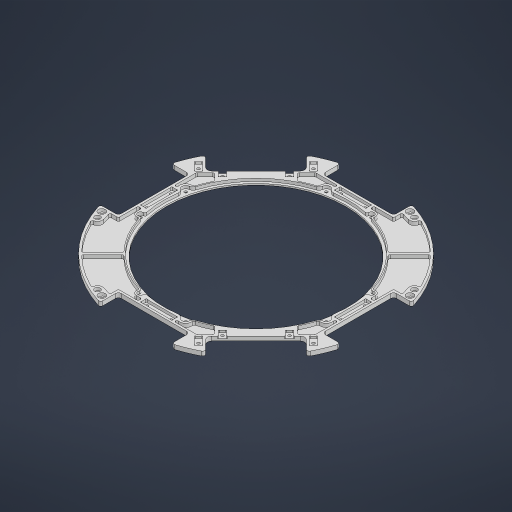
# Autodesk Inventor part: BasePlate
Saved by Autodesk Inventor 2024.2 (Build 282272000, 272)
## iProperties
Created: 2023-12-21
Part Number: BasePlate
Material: 一般
Document SubType Name: Modeling
Designer: Hanaoka
Density: 1 g/cm^3
Appearance: 既定
Author: Hanaoka
Autodesk Inventor part; units mm, degrees
ref_plane "YZ Plane" through (0, 0, 0) normal (1, 0, 0) x (0, 1, 0)
ref_plane "XZ Plane" through (0, 0, 0) normal (0, 1, 0) x (-1, 0, 0)
ref_plane "XY Plane" through (0, 0, 0) normal (0, 0, 1) x (1, 0, 0)
derived "MotorMount_main.ipt"
sketch "スケッチ4" plane through (-11, -15, 0) normal (0, -1, 0) x (1, 0, 0)
  circle A0 centre (19.5, 2) radius 0.8 projected
  circle A1 centre (2.5, 2) radius 0.8 projected
  line L0 (22, 0) -> (0, 0) projected
  line L1 (0, 0) -> (0, 4) projected
  line L2 (22, 4) -> (0, 4) projected
  line L3 (22, 0) -> (22, 4) projected
  circle A2 centre (11, -66) radius 90 construction
  line L4 (2.5, 2) -> (19.5, 2) construction
  line L5 (11, 2) -> (11, -66) construction
  circle A3 centre (11, -66) radius 88
  line L6 (-14, 18.3742) -> (-14, 7.5)
  line L7 (-12, 5.5) -> (34, 5.5)
  line L8 (36, 7.5) -> (36, 18.3742)
  arc A4 (-14, 7.5) -> (-12, 5.5) centre (-12, 7.5) ccw
  arc A5 (34, 5.5) -> (36, 7.5) centre (34, 7.5) ccw
  line L9 (0, 0) -> (22, 0)
  line L10 (22, 0) -> (22, 4)
  line L11 (22, 4) -> (0, 4)
  line L12 (0, 4) -> (0, 0)
  circle A6 centre (19.5, 2) radius 1
  circle A7 centre (2.5, 2) radius 1
  circle A8 centre (-57, -74.5) radius 1
  line L13 (-59, -77) -> (-55, -77)
  line L14 (-57, -74.5) -> (-57, -57.5) construction
  line L15 (-59, -55) -> (-59, -77)
  line L16 (-55, -55) -> (-59, -55)
  line L17 (-55, -77) -> (-55, -55)
  line L18 (-60.5, -89) -> (-60.5, -43)
  circle A9 centre (-57, -57.5) radius 1
  arc A10 (-62.5, -91) -> (-60.5, -89) centre (-62.5, -89) ccw
  line L19 (-62.5, -41) -> (-73.3742, -41)
  arc A11 (-60.5, -43) -> (-62.5, -41) centre (-62.5, -43) ccw
  line L20 (-73.3742, -91) -> (-62.5, -91)
  circle A12 centre (19.5, -134) radius 1
  line L21 (22, -136) -> (22, -132)
  line L22 (19.5, -134) -> (2.5, -134) construction
  line L23 (0, -136) -> (22, -136)
  line L24 (0, -132) -> (0, -136)
  line L25 (22, -132) -> (0, -132)
  line L26 (34, -137.5) -> (-12, -137.5)
  circle A13 centre (2.5, -134) radius 1
  arc A14 (36, -139.5) -> (34, -137.5) centre (34, -139.5) ccw
  line L27 (-14, -139.5) -> (-14, -150.3742)
  arc A15 (-12, -137.5) -> (-14, -139.5) centre (-12, -139.5) ccw
  line L28 (36, -150.3742) -> (36, -139.5)
  circle A16 centre (79, -57.5) radius 1
  line L29 (81, -55) -> (77, -55)
  line L30 (79, -57.5) -> (79, -74.5) construction
  line L31 (81, -77) -> (81, -55)
  line L32 (77, -77) -> (81, -77)
  line L33 (77, -55) -> (77, -77)
  line L34 (82.5, -43) -> (82.5, -89)
  circle A17 centre (79, -74.5) radius 1
  arc A18 (84.5, -41) -> (82.5, -43) centre (84.5, -43) ccw
  line L35 (84.5, -91) -> (95.3742, -91)
  arc A19 (82.5, -89) -> (84.5, -91) centre (84.5, -89) ccw
  line L36 (95.3742, -41) -> (84.5, -41)
  arc A20 (77.7071, -55) -> (77, -55.7071) centre (77.3536, -55.3536) ccw
  line L37 (77.3536, -55.3536) -> (77.3536, -55) construction
  line L38 (77.3536, -55.3536) -> (77, -55.3536) construction
  line L39 (77.3536, -55.3536) -> (77, -55) construction
  line L40 (80.6464, -55) -> (80.6464, -55.3536) construction
  line L41 (80.6464, -55.3536) -> (81, -55.3536) construction
  line L42 (77.3536, -77) -> (77.3536, -76.6464) construction
  line L43 (77.3536, -76.6464) -> (77, -76.6464) construction
  line L44 (81, -76.6464) -> (80.6464, -76.6464) construction
  line L45 (80.6464, -76.6464) -> (80.6464, -77) construction
  line L46 (81, -77) -> (80.6464, -76.6464) construction
  line L47 (77.3536, -76.6464) -> (77, -77) construction
  line L48 (81, -55) -> (80.6464, -55.3536) construction
  arc A21 (81, -55.7071) -> (80.2929, -55) centre (80.6464, -55.3536) ccw
  arc A22 (80.2929, -77) -> (81, -76.2929) centre (80.6464, -76.6464) ccw
  arc A23 (77, -76.2929) -> (77.7071, -77) centre (77.3536, -76.6464) ccw
  arc A24 (21.2929, 0) -> (22, 0.7071) centre (21.6464, 0.3536) ccw
  arc A25 (22, 3.2929) -> (21.2929, 4) centre (21.6464, 3.6464) ccw
  arc A26 (0, 0.7071) -> (0.7071, 0) centre (0.3536, 0.3536) ccw
  arc A27 (0.7071, 4) -> (0, 3.2929) centre (0.3536, 3.6464) ccw
  arc A28 (-55, -55.7071) -> (-55.7071, -55) centre (-55.3536, -55.3536) ccw
  arc A29 (-58.2929, -55) -> (-59, -55.7071) centre (-58.6464, -55.3536) ccw
  arc A30 (-55.7071, -77) -> (-55, -76.2929) centre (-55.3536, -76.6464) ccw
  arc A31 (-59, -76.2929) -> (-58.2929, -77) centre (-58.6464, -76.6464) ccw
  arc A32 (0.7071, -132) -> (0, -132.7071) centre (0.3536, -132.3536) ccw
  arc A33 (0, -135.2929) -> (0.7071, -136) centre (0.3536, -135.6464) ccw
  arc A34 (22, -132.7071) -> (21.2929, -132) centre (21.6464, -132.3536) ccw
  arc A35 (21.2929, -136) -> (22, -135.2929) centre (21.6464, -135.6464) ccw
  point P0 (11, 0)
  point P1 (-14, 5.5)
  point P2 (36, 5.5)
  point P3 (-57, -66)
  point P4 (-60.5, -91)
  point P5 (-60.5, -41)
  point P6 (11, -134)
  point P7 (36, -137.5)
  point P8 (-14, -137.5)
  point P9 (79, -66)
  point P10 (82.5, -41)
  point P11 (82.5, -91)
  point P12 (22, -135.2929)
  point P13 (21.2929, -136)
  point P14 (0.7071, -136)
  point P15 (0, -135.2929)
  point P16 (0, -132.7071)
  point P17 (0.7071, -132)
  point P18 (21.2929, -132)
  point P19 (22, -132.7071)
  point P20 (-58.2929, -77)
  point P21 (-59, -76.2929)
  point P22 (-59, -55.7071)
  point P23 (-58.2929, -55)
  point P24 (-55.7071, -55)
  point P25 (-55, -55.7071)
  point P26 (-55, -76.2929)
  point P27 (-55.7071, -77)
  point P28 (0, 3.2929)
  point P29 (0.7071, 4)
  point P30 (21.2929, 4)
  point P31 (22, 3.2929)
  point P32 (22, 0.7071)
  point P33 (21.2929, 0)
  point P34 (0.7071, 0)
  point P35 (0, 0.7071)
  dimension "d4" = 180
  dimension "d5" = 68
  dimension "d6" = 176
  dimension "d11" = 1.5
  dimension "d12" = 50
  dimension "d13" = 2
  dimension "d14" = 2
  dimension "d17" = 360
  dimension "d31" = 0.5
  dimension "d32" = 0.5
  dimension "d35" = 360
  constraints: 90 end point, 50 point on circle, 34 centre point, 32 point on line, 13 coincident, 8 equal length, 6 perpendicular, 5 equal radius, 4 horizontal, 4 tangent, 4 vertical, 3 parallel, 1 midpoint, 190 other
  measures "d4" diameter of A2
  measures "d5" distance of L5.start L5.end
  measures "d6" diameter of A3
  measures "d11" distance between parallel lines of L7 L2
  measures "d12" distance of point (-14, 5.5) point (36, 5.5)
  measures "d13" radius of A4
  measures "d14" diameter of A7
  measures "d31" radius of A20
  measures "d32" distance of L37.start L29.end
extrude "押し出し2" add sketch "スケッチ4" along normal blind 1 contours A24 L0 | L0 L1 L2 L3 | L3 A24 | A26 L0 | L3 A25 | A26 L1 | L2 A25 | A27 L1 | L2 A27 | L36 A18 L34 A19 L35 A3 L28 A14 L26 A15 L27 L20 A10 L18 A11 L19 L6 A4 L7 A5 L8 | L15 L16 L17 L13 | A31 L15 | L13 A31 | L13 A30 | A29 L15 | L17 A30 | A29 L16 | L17 A28 | A28 L16 | L23 L24 L25 L21 | A35 L23 | L21 A35 | L21 A34 | A33 L23 | L25 A34 | A33 L24 | L25 A32 | A32 L24 | L31 L32 L33 L29 | A21 L31 | L29 A21 | L29 A20 | A22 L31 | L33 A20 | A22 L32 | L33 A23 | A23 L32
extrude "押し出し3" add sketch "スケッチ4" against normal blind 2 contours L36 A18 L34 A19 L35 A3 L28 A14 L26 A15 L27 L20 A10 L18 A11 L19 L6 A4 L7 A5 L8
fillet "フィレット1" radius 1.5 8 edges at (-84.3742, -14.5, -41) (-25, -14.5, 18.3742) (25, -14.5, 18.3742) (84.3742, -14.5, -41) (84.3742, -14.5, -91) (25, -14.5, -150.3742) (-25, -14.5, -150.3742) (-84.3742, -14.5, -91)
sketch "溝切り" plane through (-23, -13, 5.5) normal (0, 1, 0) x (1, 0, 0)
  circle A0 centre (102.5487, 100) radius 2.5
  line L0 (96.5, 96.5) -> (105.3408, 96.5) projected
  arc A1 (106.7686, 98.4595) -> (49.9595, 155.2686) centre (23, 71.5) ccw projected
  circle A2 centre (102.5487, 100) radius 3.5 construction
  line L1 (85.2254, 133.7254) -> (-39.2254, 9.2746) construction
  arc A3 (-60.7686, 44.5405) -> (-3.9595, -12.2686) centre (23, 71.5) ccw projected
  circle A4 centre (51.5, 151.0487) radius 2.5
  circle A5 centre (51.5, 151.0487) radius 3.5 construction
  line L2 (-39.2254, 133.7254) -> (85.2254, 9.2746) construction
  arc A6 (49.9595, -12.2686) -> (106.7686, 44.5405) centre (23, 71.5) ccw projected
  arc A7 (-3.9595, 155.2686) -> (-60.7686, 98.4595) centre (23, 71.5) ccw projected
  circle A8 centre (-5.5, -8.0487) radius 2.5
  circle A9 centre (-5.5, -8.0487) radius 3.5 construction
  circle A10 centre (-56.5487, 43) radius 3.5 construction
  circle A11 centre (-56.5487, 43) radius 2.5
  circle A12 centre (102.5487, 100) radius 1.3
  circle A13 centre (51.5, 151.0487) radius 1.3
  circle A14 centre (-56.5487, 43) radius 1.3
  circle A15 centre (-5.5, -8.0487) radius 1.3
  circle A16 centre (23, 71.5) radius 63
  line L3 (-54.3392, 113.4839) -> (-46.9146, 106.0593)
  line L4 (-42.672, 106.0593) -> (-11.5593, 137.172)
  line L5 (-11.5593, 141.4146) -> (-18.9839, 148.8392)
  arc A17 (-46.9146, 106.0593) -> (-42.672, 106.0593) centre (-44.7933, 108.1806) ccw
  arc A18 (-11.5593, 137.172) -> (-11.5593, 141.4146) centre (-13.6806, 139.2933) ccw
  circle A19 centre (-41.9648, 136.4648) radius 21 construction
  line L6 (64.9839, -5.8392) -> (57.5593, 1.5854)
  line L7 (57.5593, 5.828) -> (88.672, 36.9407)
  line L8 (92.9146, 36.9407) -> (100.3392, 29.5161)
  arc A20 (57.5593, 5.828) -> (57.5593, 1.5854) centre (59.6806, 3.7067) ccw
  arc A21 (92.9146, 36.9407) -> (88.672, 36.9407) centre (90.7933, 34.8194) ccw
  circle A22 centre (8.2095, 135.5648) radius 2.75 construction
  circle A23 centre (8.2095, 135.5648) radius 1
  line L9 (8.2095, 135.5648) -> (23, 71.5) construction
  arc A24 (10.889, 136.1834) -> (5.53, 134.9462) centre (8.2095, 135.5648) ccw
  line L10 (5.53, 134.9462) -> (6.1621, 132.2082)
  line L11 (10.889, 136.1834) -> (11.5211, 133.4454)
  circle A25 centre (-41.0648, 86.2905) radius 2.75 construction
  circle A26 centre (-41.0648, 86.2905) radius 1
  arc A27 (-40.4462, 88.97) -> (-41.6834, 83.611) centre (-41.0648, 86.2905) ccw
  line L12 (-40.4462, 88.97) -> (-37.7082, 88.3379)
  line L13 (-41.6834, 83.611) -> (-38.9454, 82.9789)
  circle A28 centre (87.0648, 56.7095) radius 2.75 construction
  circle A29 centre (87.0648, 56.7095) radius 1
  arc A30 (86.4462, 54.03) -> (87.6834, 59.389) centre (87.0648, 56.7095) ccw
  line L14 (86.4462, 54.03) -> (83.7082, 54.6621)
  line L15 (87.6834, 59.389) -> (84.9454, 60.0211)
  line L16 (35.111, 6.8166) -> (34.4789, 9.5546)
  line L17 (40.47, 8.0538) -> (39.8379, 10.7918)
  circle A31 centre (37.7905, 7.4352) radius 2.75 construction
  circle A32 centre (37.7905, 7.4352) radius 1
  arc A33 (35.111, 6.8166) -> (40.47, 8.0538) centre (37.7905, 7.4352) ccw
  circle A34 centre (23, 71.5) radius 64
  line L18 (-48.5, 94.5) -> (-48.5, 96.331) construction
  line L19 (-48.5, 96.331) -> (-58.019, 105.85) construction
  line L20 (-48.5, 94.5) -> (-48.5, 48.5) projected
  line L21 (0, 143) -> (-1.831, 143) construction
  line L22 (-1.831, 143) -> (-11.35, 152.519) construction
  arc A35 (-60.7686, 98.4595) -> (-59.3408, 96.5) centre (-59.3408, 98) ccw projected
  line L23 (-59.3408, 96.5) -> (-50.5, 96.5) projected
  arc A36 (-48.5, 94.5) -> (-50.5, 96.5) centre (-50.5, 94.5) ccw projected
  arc A37 (-2, 153.8408) -> (-3.9595, 155.2686) centre (-3.5, 153.8408) ccw projected
  line L24 (-2, 145) -> (-2, 153.8408) projected
  arc A38 (-2, 145) -> (0, 143) centre (0, 145) ccw projected
  line L25 (46, 143) -> (0, 143) projected
  point P0 (23, 5.5)
  point P1 (-44.7933, 103.9379)
  point P2 (-9.4379, 139.2933)
  point P3 (100.3392, 29.5161)
  point P4 (39.8379, 10.7918)
  point P5 (34.4789, 9.5546)
  point P6 (84.9454, 60.0211)
  point P7 (83.7082, 54.6621)
  point P8 (-38.9454, 82.9789)
  point P9 (-37.7082, 88.3379)
  point P10 (-39.9207, 83.2041)
  point P11 (34.7041, 8.5793)
  point P12 (40.0631, 9.8165)
  point P13 (84.6835, 54.4369)
  point P14 (85.9207, 59.7959)
  point P15 (11.2959, 134.4207)
  point P16 (5.9369, 133.1835)
  point P17 (-38.6835, 88.5631)
  point P18 (-50.6269, 109.7716)
  point P19 (-11.35, 152.519)
  dimension "d20" = 5
  dimension "d22" = 7
  dimension "d23" = 2.6
  dimension "d37" = 50
  dimension "d38" = 3
  dimension "d39" = 42
  dimension "d40" = 13.5
  dimension "d45" = 2
  dimension "d46" = 5.5
  dimension "d47" = 32
  dimension "d102" = 8
  dimension "d106" = 126
  dimension "d107" = 1
  constraints: 42 end point, 38 symmetric about line, 31 centre point, 25 point on circle, 18 coincident, 11 tangent, 7 parallel, 5 equal radius, 5 point on line, 2 midpoint, 1 collinear, 1 vertical, 17 other
  measures "d20" diameter of A0
  measures "d22" diameter of A2
  measures "d23" diameter of A12
  measures "d37" distance of point (-44.793, 103.938) point (-9.438, 139.293)
  measures "d38" radius of A17
  measures "d39" diameter of A19
  measures "d40" distance from line of L5.end L4
  measures "d45" diameter of A23
  measures "d46" diameter of A22
  measures "d47" angle of L2 L9
  measures "d102" distance from line of point (-50.627, 109.772) L19
  measures "d106" diameter of A16
  measures "d107" radial gap between concentric circles of A16 A34
extrude "押し出し4" cut sketch "溝切り" against normal up to surface (3 mm away) contours A12 | A13 | A14 | A15
extrude "押し出し5" cut sketch "溝切り" against normal blind 2 contours A0 | A4 | A8 | A11 | A15 | A16 | A16 L11 A34 L15 | A16 L10 A34 L11 | L15 A34 L14 A16 | A16 L12 A34 L10 | A34 L10 A24 L11 | L14 A34 L17 A16 | L15 A30 L14 A34 | A16 L13 A34 L12 | L17 A34 L16 A16 | A16 L16 A34 L13 | A34 L13 A27 L12 | L17 A33 L16 A34
extrude "押し出し6" cut sketch "溝切り" against normal up to surface (3 mm away) contours L6 A20 L7 A21 L8 A6 | L5 A18 L4 A17 L3 A7 | A16 | A23 | A26 | A29 | A32
fillet "フィレット2" radius 1.5 12 edges at (-77.3392, -14.5, -107.9839) (-41.9839, -14.5, -143.3392) (41.9839, -14.5, 11.3392) (77.3392, -14.5, -24.0161) (-62.9207, -14, -77.7041) (-61.6835, -14, -83.0631) (11.7041, -14, -3.0793) (17.0631, -14, -4.3165) (61.6835, -14, -48.9369) (62.9207, -14, -54.2959) (-17.0631, -14, -127.6835) (-11.7041, -14, -128.9207)
sketch "シャフト用はめ穴" plane through (-23, -13, -137.5) normal (0, 1, 0) x (1, 0, 0)
  circle A0 centre (-54.5262, -105.1146) radius 1
  circle A1 centre (-54.5262, -105.1146) radius 2
  circle A2 centre (-41.4205, -88) radius 2
  circle A3 centre (-41.4205, -88) radius 1
  circle A4 centre (-56.5487, -100) radius 2.5 projected
  circle A5 centre (23, -71.5) radius 63 projected
  arc A6 (-56.5487, -100) -> (-54.5262, -105.1146) centre (23, -71.5) ccw construction
  line L0 (85.2254, -9.2746) -> (-39.2254, -133.7254) construction
  line L1 (-39.2254, -9.2746) -> (85.2254, -133.7254) construction
  circle A7 centre (-10.6146, -149.0262) radius 1
  circle A8 centre (-10.6146, -149.0262) radius 2
  circle A9 centre (-41.4205, -88) radius 2.5 construction
  arc A10 (5.9369, -9.8165) -> (-38.6835, -54.4369) centre (23, -71.5) ccw projected
  line L2 (-43.7071, -82.5) -> (-46.2929, -82.5) projected
  circle A11 centre (6.5, -135.9205) radius 2
  circle A12 centre (6.5, -135.9205) radius 1
  circle A13 centre (6.5, -135.9205) radius 2.5 construction
  circle A14 centre (56.6146, 6.0262) radius 1
  circle A15 centre (56.6146, 6.0262) radius 2
  circle A16 centre (39.5, -7.0795) radius 2
  circle A17 centre (39.5, -7.0795) radius 1
  circle A18 centre (100.5262, -37.8854) radius 1
  circle A19 centre (100.5262, -37.8854) radius 2
  circle A20 centre (87.4205, -55) radius 2
  circle A21 centre (87.4205, -55) radius 1
  line L3 (23, -71.5) -> (-41.4205, -88) construction
  point P0 (23, -137.5)
  point P1 (33.5618, -134.6225)
  point P2 (-40.1225, -60.9382)
  dimension "d50" = 2
  dimension "d51" = 4
  dimension "d52" = 1
  dimension "d53" = 5
  dimension "d54" = 3
  constraints: 19 centre point, 13 symmetric about line, 12 coincident, 2 end point, 2 equal radius, 2 midpoint, 2 point on circle, 1 tangent, 13 other
  measures "d50" diameter of A0
  measures "d51" diameter of A1
  measures "d53" diameter of A9
  measures "d54" distance edge to line of A9 L2
extrude "押し出し7" cut sketch "シャフト用はめ穴" against normal up to surface (2 mm away) contours A0 | A1 | A2 | A3 | A7 | A8 | A11 | A12 | A14 | A15 | A16 | A17 | A18 | A19 | A20 | A21
extrude "押し出し8" cut sketch "シャフト用はめ穴" against normal up to surface (3 mm away) contours A0 | A3 | A7 | A12 | A14 | A17 | A18 | A21
sketch "キッカー用はめあい" plane through (-23, -13, -137.5) normal (0, 1, 0) x (1, 0, 0)
  circle A0 centre (83.1212, -108.0745) radius 1
  circle A1 centre (59.5745, -131.6212) radius 1
  line L0 (88.672, -106.0593) -> (57.5593, -137.172) projected
  line L1 (73.1156, -121.6156) -> (68.2548, -116.7548) construction
  line L2 (57.5593, -137.172) -> (88.672, -106.0593) projected
  arc A2 (5.9369, -9.8165) -> (-38.6835, -54.4369) centre (23, -71.5) ccw projected
  line L3 (59.5745, -131.6212) -> (83.1212, -108.0745) construction
  line L4 (86.3031, -108.4281) -> (82.7676, -104.8925)
  line L5 (82.7676, -104.8925) -> (79.9392, -107.721)
  line L6 (79.9392, -107.721) -> (83.4747, -111.2565)
  circle A3 centre (83.1212, -108.0745) radius 2 construction
  line L7 (59.9281, -134.8031) -> (56.3925, -131.2676)
  line L8 (56.3925, -131.2676) -> (59.221, -128.4392)
  line L9 (59.221, -128.4392) -> (62.7565, -131.9747)
  line L10 (82.7676, -104.8925) -> (83.1212, -105.2461)
  line L11 (79.9392, -107.721) -> (80.2927, -108.0745)
  line L12 (-21.5477, -116.0477) -> (67.5477, -26.9523) construction
  circle A4 centre (23, -71.5) radius 63 projected
  circle A5 centre (-13.5745, -11.3788) radius 1
  circle A6 centre (-37.1212, -34.9255) radius 1
  line L13 (-27.1156, -21.3844) -> (-22.2548, -26.2452) construction
  line L14 (-37.1212, -34.9255) -> (-13.5745, -11.3788) construction
  line L15 (-13.9281, -8.1969) -> (-10.3925, -11.7324)
  line L16 (-10.3925, -11.7324) -> (-13.221, -14.5608)
  line L17 (-13.221, -14.5608) -> (-16.7565, -11.0253)
  circle A7 centre (-13.5745, -11.3788) radius 2 construction
  line L18 (-40.3031, -34.5719) -> (-36.7676, -38.1075)
  line L19 (-36.7676, -38.1075) -> (-33.9392, -35.279)
  line L20 (-33.9392, -35.279) -> (-37.4747, -31.7435)
  line L21 (-10.3925, -11.7324) -> (-10.7461, -11.3788)
  line L22 (-13.221, -14.5608) -> (-13.5745, -14.2073)
  line L23 (-40.3031, -34.5719) -> (-37.4747, -31.7435)
  line L24 (-42.672, -36.9407) -> (-11.5593, -5.828) projected
  line L25 (-16.7565, -11.0253) -> (-13.9281, -8.1969)
  line L26 (-54.3392, -37.2943) -> (-51.5108, -34.4659)
  line L27 (-51.5108, -34.4659) -> (-45.8539, -40.1227)
  line L28 (-45.8539, -40.1227) -> (-48.6824, -42.9512)
  line L29 (-48.6824, -42.9512) -> (-54.3392, -37.2943)
  line L30 (-46.9146, -36.9407) -> (-52.9014, -30.954) projected
  line L31 (-11.5593, -5.828) -> (-42.672, -36.9407) projected
  circle A8 centre (-50.0966, -38.7085) radius 1
  line L32 (-51.5108, -40.1227) -> (-48.6824, -37.2943) construction
  line L33 (-47.2681, -41.5369) -> (-52.925, -35.8801) construction
  arc A9 (-53.8392, -36.7943) -> (-53.8392, -37.7943) centre (-53.8392, -37.2943) ccw
  line L34 (-54.3392, -37.2943) -> (-53.8392, -37.2943) construction
  line L35 (-53.8392, -37.2943) -> (-54.0892, -37.0443) construction
  line L36 (-53.8392, -37.2943) -> (-54.0892, -37.5443) construction
  arc A10 (-51.0108, -34.9659) -> (-52.0108, -34.9659) centre (-51.5108, -34.9659) ccw
  arc A11 (-49.1824, -42.4512) -> (-48.1824, -42.4512) centre (-48.6824, -42.4512) ccw
  arc A12 (-46.3539, -40.6227) -> (-46.3539, -39.6227) centre (-46.3539, -40.1227) ccw
  line L37 (-11.2057, 5.8392) -> (-14.0341, 3.0108)
  line L38 (-14.0341, 3.0108) -> (-8.3773, -2.6461)
  line L39 (-8.3773, -2.6461) -> (-5.5488, 0.1824)
  line L40 (-5.5488, 0.1824) -> (-11.2057, 5.8392)
  circle A13 centre (-9.7915, 1.5966) radius 1
  arc A14 (-10.7057, 5.3392) -> (-11.7057, 5.3392) centre (-11.2057, 5.3392) ccw
  arc A15 (-13.5341, 3.5108) -> (-13.5341, 2.5108) centre (-13.5341, 3.0108) ccw
  arc A16 (-6.0488, -0.3176) -> (-6.0488, 0.6824) centre (-6.0488, 0.1824) ccw
  arc A17 (-8.8773, -2.1461) -> (-7.8773, -2.1461) centre (-8.3773, -2.1461) ccw
  line L41 (57.2057, -148.8392) -> (60.0341, -146.0108)
  line L42 (60.0341, -146.0108) -> (54.3773, -140.3539)
  line L43 (54.3773, -140.3539) -> (51.5488, -143.1824)
  line L44 (51.5488, -143.1824) -> (57.2057, -148.8392)
  circle A18 centre (55.7915, -144.5966) radius 1
  arc A19 (56.7057, -148.3392) -> (57.7057, -148.3392) centre (57.2057, -148.3392) ccw
  arc A20 (59.5341, -146.5108) -> (59.5341, -145.5108) centre (59.5341, -146.0108) ccw
  arc A21 (52.0488, -142.6824) -> (52.0488, -143.6824) centre (52.0488, -143.1824) ccw
  arc A22 (54.8773, -140.8539) -> (53.8773, -140.8539) centre (54.3773, -140.8539) ccw
  line L45 (94.6824, -100.0488) -> (100.3392, -105.7057)
  arc A23 (99.8392, -106.2057) -> (99.8392, -105.2057) centre (99.8392, -105.7057) ccw
  line L46 (100.3392, -105.7057) -> (97.5108, -108.5341)
  arc A24 (97.0108, -108.0341) -> (98.0108, -108.0341) centre (97.5108, -108.0341) ccw
  line L47 (97.5108, -108.5341) -> (91.8539, -102.8773)
  circle A25 centre (96.0966, -104.2915) radius 1
  line L48 (91.8539, -102.8773) -> (94.6824, -100.0488)
  arc A26 (95.1824, -100.5488) -> (94.1824, -100.5488) centre (94.6824, -100.5488) ccw
  arc A27 (92.3539, -102.3773) -> (92.3539, -103.3773) centre (92.3539, -102.8773) ccw
  arc A28 (83.2676, -105.3925) -> (82.2676, -105.3925) centre (82.7676, -105.3925) ccw
  line L49 (82.5176, -105.1425) -> (82.7676, -105.3925) construction
  line L50 (82.7676, -105.3925) -> (83.0176, -105.1425) construction
  line L51 (82.7676, -105.3925) -> (82.7676, -104.8925) construction
  line L52 (80.1892, -107.971) -> (80.4392, -107.721) construction
  line L53 (80.4392, -107.721) -> (80.1892, -107.471) construction
  line L54 (80.4392, -107.721) -> (79.9392, -107.721) construction
  arc A29 (80.4392, -107.221) -> (80.4392, -108.221) centre (80.4392, -107.721) ccw
  arc A30 (56.8925, -130.7676) -> (56.8925, -131.7676) centre (56.8925, -131.2676) ccw
  arc A31 (59.721, -128.9392) -> (58.721, -128.9392) centre (59.221, -128.9392) ccw
  arc A32 (-10.8925, -12.2324) -> (-10.8925, -11.2324) centre (-10.8925, -11.7324) ccw
  arc A33 (-13.721, -14.0608) -> (-12.721, -14.0608) centre (-13.221, -14.0608) ccw
  arc A34 (-34.4392, -35.779) -> (-34.4392, -34.779) centre (-34.4392, -35.279) ccw
  arc A35 (-37.2676, -37.6075) -> (-36.2676, -37.6075) centre (-36.7676, -37.6075) ccw
  point P0 (23, -137.5)
  point P1 (84.3641, -89.6782)
  point P2 (41.1782, -132.8641)
  point P3 (86.3031, -108.4281)
  point P4 (83.4966, -105.6216)
  point P5 (80.6463, -108.4281)
  point P6 (-11.1216, -11.0034)
  point P7 (-13.9281, -13.8537)
  point P8 (95.1824, -100.5488)
  point P9 (94.1824, -100.5488)
  point P10 (92.3539, -102.3773)
  point P11 (92.3539, -103.3773)
  point P12 (97.0108, -108.0341)
  point P13 (98.0108, -108.0341)
  point P14 (53.8773, -140.8539)
  point P15 (52.0488, -142.6824)
  point P16 (52.0488, -143.6824)
  point P17 (59.5341, -146.5108)
  point P18 (59.5341, -145.5108)
  point P19 (54.8773, -140.8539)
  point P20 (-7.8773, -2.1461)
  point P21 (-6.0488, -0.3176)
  point P22 (-6.0488, 0.6824)
  point P23 (-13.5341, 3.5108)
  point P24 (-13.5341, 2.5108)
  point P25 (-8.8773, -2.1461)
  point P26 (-48.1824, -42.4512)
  point P27 (-46.3539, -40.6227)
  point P28 (-46.3539, -39.6227)
  point P29 (-51.0108, -34.9659)
  point P30 (-52.0108, -34.9659)
  point P31 (-49.1824, -42.4512)
  point P32 (-34.4392, -34.779)
  point P33 (-36.2676, -37.6075)
  point P34 (-37.2676, -37.6075)
  point P35 (-13.721, -14.0608)
  point P36 (-12.721, -14.0608)
  point P37 (-10.3925, -11.7324)
  point P38 (-10.3925, -11.7324)
  point P39 (-10.8925, -11.2324)
  point P40 (59.721, -128.9392)
  point P41 (58.721, -128.9392)
  point P42 (56.8925, -131.7676)
  dimension "d59" = 2
  dimension "d60" = 33.3
  dimension "d61" = 2.5
  dimension "d62" = 4
  dimension "d63" = 5
  dimension "d84" = 8
  dimension "d85" = 4
  dimension "d86" = 1.5
  dimension "d88" = 2
  dimension "d89" = 0.5
  dimension "d90" = 0.5
  dimension "d103" = 0.5
  dimension "d104" = 0.5
  constraints: 102 symmetric about line, 100 end point, 53 point on circle, 37 point on line, 34 centre point, 9 perpendicular, 7 midpoint, 7 parallel, 6 coincident, 3 equal length, 2 collinear, 2 horizontal, 2 tangent, 1 equal radius, 1 vertical, 28 other
  measures "d59" diameter of A0
  measures "d60" distance of L3.start L3.end
  measures "d61" distance between parallel lines of L0 L3
  measures "d62" diameter of A3
  measures "d63" distance of L4.start L4.end
  measures "d84" distance of L28.end L29.end
  measures "d85" distance of L26.start L26.end
  measures "d86" distance between parallel lines of L30 L27
  measures "d88" diameter of A8
  measures "d89" distance of L26.start L34.end
  measures "d90" radius of A9
  measures "d103" distance of L49.end L4.end
  measures "d104" distance of L52.end L5.end
extrude "押し出し9" cut sketch "キッカー用はめあい" against normal blind 1.5 contours A0 | A1 | L0 L6 L5 L4 | L4 A28 | A29 L6 | L5 A28 | A29 L5 | L0 L7 L8 L9 | L9 A31 | A30 L7 | L8 A31 | A30 L8 | A5 | A6 | L15 L16 L17 L24 | A32 L15 | A32 L16 | L17 A33 | L16 A33 | L23 L20 L19 L18 | L18 A35 | L19 A35 | A34 L20 | A34 L19 | A9 L26 | L26 L27 L28 L29 | L29 A9 | A10 L26 | L29 A11 | A10 L27 | L28 A11 | A12 L27 | L28 A12 | A8 | L40 L39 L38 L37 | A14 L40 | L37 A14 | L37 A15 | A16 L40 | L38 A15 | A16 L39 | L38 A17 | A17 L39 | A13 | L44 L43 L42 L41 | A19 L44 | L41 A19 | L41 A20 | A21 L44 | L42 A20 | A21 L43 | L42 A22 | A22 L43 | A18 | A26 L45 | L45 L46 L47 L48 | L48 A26 | A23 L45 | L48 A27 | A23 L46 | L47 A27 | A24 L46 | L47 A24 | A25
extrude "押し出し10" cut sketch "キッカー用はめあい" against normal up to surface (3 mm away) contours A0 | A1 | A5 | A6 | A8 | A13 | A18 | A25
fillet "フィレット4" radius 0.5 8 edges at (36.9281, -13.75, -2.6969) (39.7565, -13.75, -5.5253) (60.4747, -13.75, -26.2435) (63.3031, -13.75, -29.0719) (-63.3031, -13.75, -102.9281) (-60.4747, -13.75, -105.7565) (-39.7565, -13.75, -126.4747) (-36.9281, -13.75, -129.3031)
sketch "肉抜き" plane through (-23, -13, 5.5) normal (0, 1, 0) x (1, 0, 0)
  circle A0 centre (102.5487, 100) radius 2.5 projected
  circle A1 centre (-5.5, -8.0487) radius 2.5 projected
  circle A2 centre (51.5, 151.0487) radius 2.5 projected
  circle A3 centre (-56.5487, 43) radius 2.5 projected
  arc A4 (35.111, 6.8166) -> (40.47, 8.0538) centre (37.7905, 7.4352) ccw projected
  arc A5 (4.5872, 132.7941) -> (-38.2941, 89.9128) centre (23, 71.5) ccw projected
  arc A6 (-40.4462, 88.97) -> (-41.6834, 83.611) centre (-41.0648, 86.2905) ccw projected
  arc A7 (-40.1624, 81.8203) -> (33.3203, 8.3376) centre (23, 71.5) ccw projected
  arc A8 (10.889, 136.1834) -> (5.53, 134.9462) centre (8.2095, 135.5648) ccw projected
  arc A9 (41.4128, 10.2059) -> (84.2941, 53.0872) centre (23, 71.5) ccw projected
  arc A10 (86.4462, 54.03) -> (87.6834, 59.389) centre (87.0648, 56.7095) ccw projected
  arc A11 (86.1624, 61.1797) -> (12.6797, 134.6624) centre (23, 71.5) ccw projected
  arc A12 (34, 140.7929) -> (33.2929, 141.5) centre (33.6464, 141.1464) ccw projected
  line L0 (34, 140.7929) -> (34, 138.2071) projected
  arc A13 (33.2929, 137.5) -> (34, 138.2071) centre (33.6464, 137.8536) ccw projected
  line L1 (33.2929, 137.5) -> (12.7071, 137.5) projected
  arc A14 (12, 138.2071) -> (12.7071, 137.5) centre (12.3536, 137.8536) ccw projected
  line L2 (12, 138.2071) -> (12, 140.7929) projected
  arc A15 (12.7071, 141.5) -> (12, 140.7929) centre (12.3536, 141.1464) ccw projected
  line L3 (12.7071, 141.5) -> (33.2929, 141.5) projected
  arc A16 (-46.2929, 82.5) -> (-47, 81.7929) centre (-46.6464, 82.1464) ccw projected
  line L4 (-46.2929, 82.5) -> (-43.7071, 82.5) projected
  arc A17 (-43, 81.7929) -> (-43.7071, 82.5) centre (-43.3536, 82.1464) ccw projected
  line L5 (-43, 81.7929) -> (-43, 61.2071) projected
  arc A18 (-43.7071, 60.5) -> (-43, 61.2071) centre (-43.3536, 60.8536) ccw projected
  line L6 (-43.7071, 60.5) -> (-46.2929, 60.5) projected
  arc A19 (-47, 61.2071) -> (-46.2929, 60.5) centre (-46.6464, 60.8536) ccw projected
  line L7 (-47, 61.2071) -> (-47, 81.7929) projected
  arc A20 (12, 2.2071) -> (12.7071, 1.5) centre (12.3536, 1.8536) ccw projected
  line L8 (12, 2.2071) -> (12, 4.7929) projected
  arc A21 (12.7071, 5.5) -> (12, 4.7929) centre (12.3536, 5.1464) ccw projected
  line L9 (12.7071, 5.5) -> (33.2929, 5.5) projected
  arc A22 (34, 4.7929) -> (33.2929, 5.5) centre (33.6464, 5.1464) ccw projected
  line L10 (34, 4.7929) -> (34, 2.2071) projected
  arc A23 (33.2929, 1.5) -> (34, 2.2071) centre (33.6464, 1.8536) ccw projected
  line L11 (33.2929, 1.5) -> (12.7071, 1.5) projected
  arc A24 (89.7071, 82.5) -> (89, 81.7929) centre (89.3536, 82.1464) ccw projected
  line L12 (89.7071, 82.5) -> (92.2929, 82.5) projected
  arc A25 (93, 81.7929) -> (92.2929, 82.5) centre (92.6464, 82.1464) ccw projected
  line L13 (93, 81.7929) -> (93, 61.2071) projected
  arc A26 (92.2929, 60.5) -> (93, 61.2071) centre (92.6464, 60.8536) ccw projected
  line L14 (92.2929, 60.5) -> (89.7071, 60.5) projected
  arc A27 (89, 61.2071) -> (89.7071, 60.5) centre (89.3536, 60.8536) ccw projected
  line L15 (89, 61.2071) -> (89, 81.7929) projected
  circle A28 centre (-41.4205, 55) radius 2 projected
  circle A29 centre (6.5, 7.0795) radius 2 projected
  circle A30 centre (-54.5262, 37.8854) radius 2 projected
  circle A31 centre (-10.6146, -6.0262) radius 2 projected
  arc A32 (-13.5745, 135.1567) -> (-13.5745, 134.4496) centre (-13.221, 134.8031) ccw projected
  line L16 (-13.5745, 134.4496) -> (-10.8925, 131.7676) projected
  line L17 (-10.8925, 130.7676) -> (-12.721, 128.9392) projected
  line L18 (-13.721, 128.9392) -> (-16.4029, 131.6212) projected
  arc A33 (-16.4029, 131.6212) -> (-17.11, 131.6212) centre (-16.7565, 131.2676) ccw projected
  line L19 (-17.11, 131.6212) -> (-37.1212, 111.61) projected
  arc A34 (-37.1212, 111.61) -> (-37.1212, 110.9029) centre (-36.7676, 111.2565) ccw projected
  line L20 (-37.1212, 110.9029) -> (-34.4392, 108.221) projected
  line L21 (-34.4392, 107.221) -> (-36.2676, 105.3925) projected
  line L22 (-37.2676, 105.3925) -> (-39.9496, 108.0745) projected
  arc A35 (-39.9496, 108.0745) -> (-40.6567, 108.0745) centre (-40.3031, 107.721) ccw projected
  line L23 (-40.6567, 108.0745) -> (-42.672, 106.0593) projected
  arc A36 (-46.9146, 106.0593) -> (-42.672, 106.0593) centre (-44.7933, 108.1806) ccw projected
  line L24 (-46.9146, 106.0593) -> (-52.9014, 112.046) projected
  arc A37 (-52.9014, 112.046) -> (-55.2966, 111.6701) centre (-53.962, 110.9854) ccw projected
  arc A38 (-55.2966, 111.6701) -> (-60.7686, 98.4595) centre (23, 71.5) ccw projected
  line L25 (-48.5, 94.5) -> (-48.5, 48.5) projected
  arc A39 (-50.5, 46.5) -> (-48.5, 48.5) centre (-50.5, 48.5) ccw projected
  line L26 (-50.5, 46.5) -> (-59.3408, 46.5) projected
  arc A40 (-59.3408, 46.5) -> (-60.7686, 44.5405) centre (-59.3408, 45) ccw projected
  arc A41 (-60.7686, 44.5405) -> (-3.9595, -12.2686) centre (23, 71.5) ccw projected
  arc A42 (-3.9595, -12.2686) -> (-2, -10.8408) centre (-3.5, -10.8408) ccw projected
  line L27 (-2, -10.8408) -> (-2, -2) projected
  arc A43 (0, 0) -> (-2, -2) centre (0, -2) ccw projected
  line L28 (0, 0) -> (46, 0) projected
  arc A44 (48, -2) -> (46, 0) centre (46, -2) ccw projected
  line L29 (48, -2) -> (48, -10.8408) projected
  arc A45 (48, -10.8408) -> (49.9595, -12.2686) centre (49.5, -10.8408) ccw projected
  arc A46 (49.9595, -12.2686) -> (63.1701, -6.7966) centre (23, 71.5) ccw projected
  arc A47 (63.1701, -6.7966) -> (63.546, -4.4014) centre (62.4854, -5.462) ccw projected
  line L30 (63.546, -4.4014) -> (57.5593, 1.5854) projected
  arc A48 (57.5593, 5.828) -> (57.5593, 1.5854) centre (59.6806, 3.7067) ccw projected
  line L31 (57.5593, 5.828) -> (59.5745, 7.8433) projected
  arc A49 (59.5745, 7.8433) -> (59.5745, 8.5504) centre (59.221, 8.1969) ccw projected
  line L32 (59.5745, 8.5504) -> (56.8925, 11.2324) projected
  line L33 (56.8925, 12.2324) -> (58.721, 14.0608) projected
  line L34 (59.721, 14.0608) -> (62.4029, 11.3788) projected
  arc A50 (62.4029, 11.3788) -> (63.11, 11.3788) centre (62.7565, 11.7324) ccw projected
  line L35 (63.11, 11.3788) -> (83.1212, 31.39) projected
  arc A51 (83.1212, 31.39) -> (83.1212, 32.0971) centre (82.7676, 31.7435) ccw projected
  line L36 (83.1212, 32.0971) -> (80.4392, 34.779) projected
  line L37 (80.4392, 35.779) -> (82.2676, 37.6075) projected
  line L38 (83.2676, 37.6075) -> (85.9496, 34.9255) projected
  arc A52 (85.9496, 34.9255) -> (86.6567, 34.9255) centre (86.3031, 35.279) ccw projected
  line L39 (86.6567, 34.9255) -> (88.672, 36.9407) projected
  arc A53 (92.9146, 36.9407) -> (88.672, 36.9407) centre (90.7933, 34.8194) ccw projected
  line L40 (92.9146, 36.9407) -> (98.9014, 30.954) projected
  arc A54 (98.9014, 30.954) -> (101.2966, 31.3299) centre (99.962, 32.0146) ccw projected
  arc A55 (101.2966, 31.3299) -> (106.7686, 44.5405) centre (23, 71.5) ccw projected
  arc A56 (106.7686, 44.5405) -> (105.3408, 46.5) centre (105.3408, 45) ccw projected
  line L41 (105.3408, 46.5) -> (96.5, 46.5) projected
  arc A57 (94.5, 48.5) -> (96.5, 46.5) centre (96.5, 48.5) ccw projected
  line L42 (94.5, 48.5) -> (94.5, 94.5) projected
  arc A58 (96.5, 96.5) -> (94.5, 94.5) centre (96.5, 94.5) ccw projected
  line L43 (96.5, 96.5) -> (105.3408, 96.5) projected
  arc A59 (105.3408, 96.5) -> (106.7686, 98.4595) centre (105.3408, 98) ccw projected
  arc A60 (106.7686, 98.4595) -> (49.9595, 155.2686) centre (23, 71.5) ccw projected
  arc A61 (49.9595, 155.2686) -> (48, 153.8408) centre (49.5, 153.8408) ccw projected
  line L44 (48, 153.8408) -> (48, 145) projected
  arc A62 (46, 143) -> (48, 145) centre (46, 145) ccw projected
  line L45 (46, 143) -> (0, 143) projected
  arc A63 (-3.9595, 155.2686) -> (-17.1701, 149.7966) centre (23, 71.5) ccw projected
  arc A64 (-17.1701, 149.7966) -> (-17.546, 147.4014) centre (-16.4854, 148.462) ccw projected
  line L46 (-17.546, 147.4014) -> (-11.5593, 141.4146) projected
  arc A65 (-11.5593, 137.172) -> (-11.5593, 141.4146) centre (-13.6806, 139.2933) ccw projected
  line L47 (-11.5593, 137.172) -> (-13.5745, 135.1567) projected
  circle A66 centre (-41.4205, 55) radius 1 projected
  arc A67 (-44.4205, 55) -> (-40.5891, 52.1175) centre (-41.4205, 55) ccw
  circle A68 centre (6.5, 7.0795) radius 1 projected
  line L48 (-44.4205, 55) -> (-44.4205, 57.8536)
  line L49 (-45.4205, 58.8536) -> (-46, 58.8536)
  line L50 (-47, 57.8536) -> (-47, 46)
  line L51 (-24.7084, 25.2058) -> (-38.1482, 11.766)
  arc A69 (-39.3599, 51.4626) -> (-24.6875, 26.5984) centre (23, 71.5) ccw
  line L52 (-48, 45) -> (-51.6313, 45)
  arc A70 (-54.4798, 33.0405) -> (-39.5788, 11.7828) centre (23, 71.5) ccw
  circle A71 centre (-56.5487, 43) radius 4 construction
  arc A72 (-53.7934, 34.4629) -> (-51.1679, 38.8712) centre (-54.5262, 37.8854) ccw
  line L53 (-52.5908, 43.7183) -> (-51.1679, 38.8712)
  arc A73 (-60.7686, 44.5405) -> (-3.9595, -12.2686) centre (23, 71.5) ccw projected
  line L54 (-39.2254, 9.2746) -> (68.2548, 116.7548) construction
  arc A74 (-46, 58.8536) -> (-47, 57.8536) centre (-46, 57.8536) ccw
  arc A75 (-44.4205, 57.8536) -> (-45.4205, 58.8536) centre (-45.4205, 57.8536) ccw
  arc A76 (-39.3599, 51.4626) -> (-40.5891, 52.1175) centre (-40.3119, 51.1567) ccw
  arc A77 (-48, 45) -> (-47, 46) centre (-48, 46) ccw
  arc A78 (-51.6313, 45) -> (-52.5908, 43.7183) centre (-51.6313, 44) ccw
  arc A79 (-53.7934, 34.4629) -> (-54.4798, 33.0405) centre (-53.5841, 33.4851) ccw
  arc A80 (-24.7084, 25.2058) -> (-24.6875, 26.5984) centre (-25.4155, 25.9129) ccw
  arc A81 (-39.5788, 11.7828) -> (-38.1482, 11.766) centre (-38.8553, 12.4731) ccw
  arc A82 (3.6175, 7.9109) -> (6.5, 4.0795) centre (6.5, 7.0795) ccw
  line L55 (6.5, 4.0795) -> (9.3536, 4.0795)
  line L56 (10.3536, 3.0795) -> (10.3536, 2.5)
  line L57 (9.3536, 1.5) -> (-2.5, 1.5)
  line L58 (-23.2942, 23.7916) -> (-36.734, 10.3518)
  arc A83 (-21.9016, 23.8125) -> (2.9626, 9.1401) centre (23, 71.5) ccw
  line L59 (-3.5, 0.5) -> (-3.5, -3.1313)
  arc A84 (-36.7172, 8.9212) -> (-15.4595, -5.9798) centre (23, 71.5) ccw
  arc A85 (-9.6288, -2.6679) -> (-14.0371, -5.2934) centre (-10.6146, -6.0262) ccw
  line L60 (-4.7817, -4.0908) -> (-9.6288, -2.6679)
  arc A86 (9.3536, 1.5) -> (10.3536, 2.5) centre (9.3536, 2.5) ccw
  arc A87 (10.3536, 3.0795) -> (9.3536, 4.0795) centre (9.3536, 3.0795) ccw
  arc A88 (3.6175, 7.9109) -> (2.9626, 9.1401) centre (2.6567, 8.1881) ccw
  arc A89 (-2.5, 1.5) -> (-3.5, 0.5) centre (-2.5, 0.5) ccw
  arc A90 (-4.7817, -4.0908) -> (-3.5, -3.1313) centre (-4.5, -3.1313) ccw
  arc A91 (-15.4595, -5.9798) -> (-14.0371, -5.2934) centre (-15.0149, -5.0841) ccw
  arc A92 (-21.9016, 23.8125) -> (-23.2942, 23.7916) centre (-22.5871, 23.0845) ccw
  arc A93 (-36.734, 10.3518) -> (-36.7172, 8.9212) centre (-36.0269, 9.6447) ccw
  arc A94 (-57.0327, 104.3179) -> (-58.9036, 99.3216) centre (23, 71.5) ccw
  line L61 (-57.9568, 98) -> (-51.169, 98)
  line L62 (-59.3408, 96.5) -> (-50.5, 96.5) projected
  line L63 (-55.4004, 104.6456) -> (-50.4619, 99.7071)
  line L64 (-49.1824, 100.5488) -> (-53.8392, 105.2057) projected
  arc A95 (-55.4004, 104.6456) -> (-57.0327, 104.3179) centre (-56.1075, 103.9385) ccw
  arc A96 (-58.9036, 99.3216) -> (-57.9568, 98) centre (-57.9568, 99) ccw
  arc A97 (-51.169, 98) -> (-50.4619, 99.7071) centre (-51.169, 99) ccw
  arc A98 (-35.7969, 100.3647) -> (-39.4672, 91.2001) centre (23, 71.5) ccw
  line L65 (-35.9875, 101.5125) -> (-39.8353, 105.3603)
  arc A99 (-40.5436, 90.5084) -> (-45.2127, 85.3644) centre (-41.0648, 86.2905) ccw
  line L66 (-46.1887, 84.1464) -> (-46, 84.1464)
  line L67 (-47, 85.1464) -> (-47, 99.1957)
  line L68 (-46.7071, 99.9028) -> (-41.2496, 105.3603)
  line L69 (-46.9146, 106.0593) -> (-52.9014, 112.046) projected
  line L70 (-40.6567, 108.0745) -> (-42.672, 106.0593) projected
  arc A100 (-39.8353, 105.3603) -> (-41.2496, 105.3603) centre (-40.5425, 104.6532) ccw
  arc A101 (-35.7969, 100.3647) -> (-35.9875, 101.5125) centre (-36.6946, 100.8054) ccw
  arc A102 (-46.7071, 99.9028) -> (-47, 99.1957) centre (-46, 99.1957) ccw
  arc A103 (-47, 85.1464) -> (-46, 84.1464) centre (-46, 85.1464) ccw
  arc A104 (-46.1887, 84.1464) -> (-45.2127, 85.3644) centre (-46.1887, 85.1464) ccw
  arc A105 (-40.5436, 90.5084) -> (-39.4672, 91.2001) centre (-40.4209, 91.5009) ccw
  line L71 (-27.1156, 121.6156) -> (73.1156, 21.3844) construction
  line L72 (-39.2254, 9.2746) -> (85.2254, 133.7254) construction
  arc A106 (-4.8216, 153.4036) -> (-9.8179, 151.5327) centre (23, 71.5) ccw
  line L73 (-3.5, 152.4568) -> (-3.5, 145.669)
  line L74 (-10.1456, 149.9004) -> (-5.2071, 144.9619)
  arc A107 (-9.8179, 151.5327) -> (-10.1456, 149.9004) centre (-9.4385, 150.6075) ccw
  arc A108 (-3.5, 152.4568) -> (-4.8216, 153.4036) centre (-4.5, 152.4568) ccw
  arc A109 (-5.2071, 144.9619) -> (-3.5, 145.669) centre (-4.5, 145.669) ccw
  arc A110 (3.2999, 133.9672) -> (-5.8647, 130.2969) centre (23, 71.5) ccw
  line L75 (-7.0125, 130.4875) -> (-10.8603, 134.3353)
  arc A111 (9.1356, 139.7127) -> (3.9916, 135.0436) centre (8.2095, 135.5648) ccw
  line L76 (10.3536, 140.6887) -> (10.3536, 140.5)
  line L77 (9.3536, 141.5) -> (-4.6957, 141.5)
  line L78 (-5.4028, 141.2071) -> (-10.8603, 135.7496)
  arc A112 (-10.8603, 135.7496) -> (-10.8603, 134.3353) centre (-10.1532, 135.0425) ccw
  arc A113 (-7.0125, 130.4875) -> (-5.8647, 130.2969) centre (-6.3054, 131.1946) ccw
  arc A114 (-4.6957, 141.5) -> (-5.4028, 141.2071) centre (-4.6957, 140.5) ccw
  arc A115 (10.3536, 140.5) -> (9.3536, 141.5) centre (9.3536, 140.5) ccw
  arc A116 (9.1356, 139.7127) -> (10.3536, 140.6887) centre (9.3536, 140.6887) ccw
  arc A117 (3.2999, 133.9672) -> (3.9916, 135.0436) centre (2.9991, 134.9209) ccw
  arc A118 (50.8216, -10.4036) -> (55.8179, -8.5327) centre (23, 71.5) ccw
  line L79 (49.5, -9.4568) -> (49.5, -2.669)
  line L80 (56.1456, -6.9004) -> (51.2071, -1.9619)
  arc A119 (55.8179, -8.5327) -> (56.1456, -6.9004) centre (55.4385, -7.6075) ccw
  arc A120 (49.5, -9.4568) -> (50.8216, -10.4036) centre (50.5, -9.4568) ccw
  arc A121 (51.2071, -1.9619) -> (49.5, -2.669) centre (50.5, -2.669) ccw
  arc A122 (42.7001, 9.0328) -> (51.8647, 12.7031) centre (23, 71.5) ccw
  line L81 (53.0125, 12.5125) -> (56.8603, 8.6647)
  arc A123 (36.8644, 3.2873) -> (42.0084, 7.9564) centre (37.7905, 7.4352) ccw
  line L82 (35.6464, 2.3113) -> (35.6464, 2.5)
  line L83 (36.6464, 1.5) -> (50.6957, 1.5)
  line L84 (51.4028, 1.7929) -> (56.8603, 7.2504)
  arc A124 (56.8603, 7.2504) -> (56.8603, 8.6647) centre (56.1532, 7.9575) ccw
  arc A125 (53.0125, 12.5125) -> (51.8647, 12.7031) centre (52.3054, 11.8054) ccw
  arc A126 (50.6957, 1.5) -> (51.4028, 1.7929) centre (50.6957, 2.5) ccw
  arc A127 (35.6464, 2.5) -> (36.6464, 1.5) centre (36.6464, 2.5) ccw
  arc A128 (36.8644, 3.2873) -> (35.6464, 2.3113) centre (36.6464, 2.3113) ccw
  arc A129 (42.7001, 9.0328) -> (42.0084, 7.9564) centre (43.0009, 8.0791) ccw
  arc A130 (101.4004, 38.3544) -> (103.0327, 38.6821) centre (102.1075, 39.0615) ccw
  arc A131 (103.0327, 38.6821) -> (104.9036, 43.6784) centre (23, 71.5) ccw
  arc A132 (104.9036, 43.6784) -> (103.9568, 45) centre (103.9568, 44) ccw
  line L85 (103.9568, 45) -> (97.169, 45)
  arc A133 (97.169, 45) -> (96.4619, 43.2929) centre (97.169, 44) ccw
  line L86 (101.4004, 38.3544) -> (96.4619, 43.2929)
  arc A134 (85.8353, 37.6397) -> (87.2496, 37.6397) centre (86.5425, 38.3468) ccw
  line L87 (92.7071, 43.0972) -> (87.2496, 37.6397)
  arc A135 (92.7071, 43.0972) -> (93, 43.8043) centre (92, 43.8043) ccw
  line L88 (93, 57.8536) -> (93, 43.8043)
  arc A136 (93, 57.8536) -> (92, 58.8536) centre (92, 57.8536) ccw
  line L89 (92.1887, 58.8536) -> (92, 58.8536)
  arc A137 (92.1887, 58.8536) -> (91.2127, 57.6356) centre (92.1887, 57.8536) ccw
  arc A138 (86.5436, 52.4916) -> (85.4672, 51.7999) centre (86.4209, 51.4991) ccw
  arc A139 (86.5436, 52.4916) -> (91.2127, 57.6356) centre (87.0648, 56.7095) ccw
  arc A140 (81.7969, 42.6353) -> (85.4672, 51.7999) centre (23, 71.5) ccw
  line L90 (81.9875, 41.4875) -> (85.8353, 37.6397)
  arc A141 (81.7969, 42.6353) -> (81.9875, 41.4875) centre (82.6946, 42.1946) ccw
  arc A142 (42.3825, 135.0891) -> (39.5, 138.9205) centre (39.5, 135.9205) ccw
  line L91 (39.5, 138.9205) -> (36.6464, 138.9205)
  line L92 (35.6464, 139.9205) -> (35.6464, 140.5)
  line L93 (36.6464, 141.5) -> (48.5, 141.5)
  line L94 (69.2942, 119.2084) -> (82.734, 132.6482)
  arc A143 (67.9016, 119.1875) -> (43.0374, 133.8599) centre (23, 71.5) ccw
  line L95 (49.5, 142.5) -> (49.5, 146.1313)
  arc A144 (82.7172, 134.0788) -> (61.4595, 148.9798) centre (23, 71.5) ccw
  arc A145 (55.6288, 145.6679) -> (60.0371, 148.2934) centre (56.6146, 149.0262) ccw
  line L96 (50.7817, 147.0908) -> (55.6288, 145.6679)
  arc A146 (36.6464, 141.5) -> (35.6464, 140.5) centre (36.6464, 140.5) ccw
  arc A147 (35.6464, 139.9205) -> (36.6464, 138.9205) centre (36.6464, 139.9205) ccw
  arc A148 (42.3825, 135.0891) -> (43.0374, 133.8599) centre (43.3433, 134.8119) ccw
  arc A149 (48.5, 141.5) -> (49.5, 142.5) centre (48.5, 142.5) ccw
  arc A150 (50.7817, 147.0908) -> (49.5, 146.1313) centre (50.5, 146.1313) ccw
  arc A151 (61.4595, 148.9798) -> (60.0371, 148.2934) centre (61.0149, 148.0841) ccw
  arc A152 (67.9016, 119.1875) -> (69.2942, 119.2084) centre (68.5871, 119.9155) ccw
  arc A153 (82.734, 132.6482) -> (82.7172, 134.0788) centre (82.0269, 133.3553) ccw
  line L97 (91.4205, 84.1464) -> (92, 84.1464)
  arc A154 (92, 84.1464) -> (93, 85.1464) centre (92, 85.1464) ccw
  arc A155 (90.4205, 85.1464) -> (91.4205, 84.1464) centre (91.4205, 85.1464) ccw
  line L98 (90.4205, 88) -> (90.4205, 85.1464)
  arc A156 (90.4205, 88) -> (86.5891, 90.8825) centre (87.4205, 88) ccw
  line L99 (93, 85.1464) -> (93, 97)
  line L100 (94, 98) -> (97.6313, 98)
  arc A157 (94, 98) -> (93, 97) centre (94, 97) ccw
  arc A158 (97.6313, 98) -> (98.5908, 99.2817) centre (97.6313, 99) ccw
  line L101 (98.5908, 99.2817) -> (97.1679, 104.1288)
  arc A159 (99.7934, 108.5371) -> (97.1679, 104.1288) centre (100.5262, 105.1146) ccw
  arc A160 (99.7934, 108.5371) -> (100.4798, 109.9595) centre (99.5841, 109.5149) ccw
  arc A161 (100.4798, 109.9595) -> (85.5788, 131.2172) centre (23, 71.5) ccw
  arc A162 (85.5788, 131.2172) -> (84.1482, 131.234) centre (84.8553, 130.5269) ccw
  line L102 (70.7084, 117.7942) -> (84.1482, 131.234)
  arc A163 (70.7084, 117.7942) -> (70.6875, 116.4016) centre (71.4155, 117.0871) ccw
  arc A164 (85.3599, 91.5374) -> (70.6875, 116.4016) centre (23, 71.5) ccw
  arc A165 (85.3599, 91.5374) -> (86.5891, 90.8825) centre (86.3119, 91.8433) ccw
  arc A166 (-60.7686, 98.4595) -> (-59.3408, 96.5) centre (-59.3408, 98) ccw projected
  line L103 (-59.3408, 96.5) -> (-50.5, 96.5) projected
  arc A167 (-48.5, 94.5) -> (-50.5, 96.5) centre (-50.5, 94.5) ccw projected
  arc A168 (-2, 145) -> (0, 143) centre (0, 145) ccw projected
  line L104 (-2, 145) -> (-2, 153.8408) projected
  arc A169 (-2, 153.8408) -> (-3.9595, 155.2686) centre (-3.5, 153.8408) ccw projected
  arc A170 (-10.8925, 130.7676) -> (-10.8925, 131.7676) centre (-10.8925, 131.2676) ccw projected
  arc A171 (-13.721, 128.9392) -> (-12.721, 128.9392) centre (-13.221, 128.9392) ccw projected
  arc A172 (-34.4392, 107.221) -> (-34.4392, 108.221) centre (-34.4392, 107.721) ccw projected
  arc A173 (-37.2676, 105.3925) -> (-36.2676, 105.3925) centre (-36.7676, 105.3925) ccw projected
  arc A174 (56.8925, 12.2324) -> (56.8925, 11.2324) centre (56.8925, 11.7324) ccw projected
  arc A175 (59.721, 14.0608) -> (58.721, 14.0608) centre (59.221, 14.0608) ccw projected
  arc A176 (80.4392, 35.779) -> (80.4392, 34.779) centre (80.4392, 35.279) ccw projected
  arc A177 (83.2676, 37.6075) -> (82.2676, 37.6075) centre (82.7676, 37.6075) ccw projected
  line L105 (40.3828, 8.4319) -> (40.47, 8.0538) projected
  line L106 (35.111, 6.8166) -> (35.0237, 7.1946) projected
  line L107 (-41.3054, 83.5237) -> (-41.6834, 83.611) projected
  line L108 (-40.4462, 88.97) -> (-40.0681, 88.8828) projected
  line L109 (5.6172, 134.5681) -> (5.53, 134.9462) projected
  line L110 (10.889, 136.1834) -> (10.9763, 135.8054) projected
  line L111 (87.3054, 59.4763) -> (87.6834, 59.389) projected
  line L112 (86.4462, 54.03) -> (86.0681, 54.1172) projected
  arc A178 (10.9763, 135.8054) -> (12.6797, 134.6624) centre (12.4378, 136.1428) ccw projected
  arc A179 (86.1624, 61.1797) -> (87.3054, 59.4763) centre (87.6428, 60.9378) ccw projected
  arc A180 (86.0681, 54.1172) -> (84.2941, 53.0872) centre (85.7307, 52.6557) ccw projected
  arc A181 (41.4128, 10.2059) -> (40.3828, 8.4319) centre (41.8443, 8.7693) ccw projected
  arc A182 (35.0237, 7.1946) -> (33.3203, 8.3376) centre (33.5622, 6.8572) ccw projected
  arc A183 (-40.1624, 81.8203) -> (-41.3054, 83.5237) centre (-41.6428, 82.0622) ccw projected
  arc A184 (-40.0681, 88.8828) -> (-38.2941, 89.9128) centre (-39.7307, 90.3443) ccw projected
  arc A185 (4.5872, 132.7941) -> (5.6172, 134.5681) centre (4.1557, 134.2307) ccw projected
  point P0 (23, 5.5)
  point P1 (-24.0172, 25.897)
  point P2 (-38.8678, 11.0465)
  point P3 (-24.0172, 25.897)
  point P4 (-38.8678, 11.0465)
  point P5 (-56.4528, 105.698)
  point P6 (-59.3408, 98)
  point P7 (-59.3408, 98)
  point P8 (-35.4788, 101.0038)
  point P9 (-44.7344, 84.1464)
  point P10 (92.0943, 58.8491)
  point P11 (35.6509, 2.4057)
  point P12 (10.3491, 140.5943)
  point P13 (-46.0943, 84.1509)
  dimension "d71" = 1.5
  dimension "d72" = 3
  dimension "d73" = 1.5
  dimension "d74" = 1.5
  dimension "d75" = 1.5
  dimension "d76" = 8
  dimension "d77" = 1.5
  dimension "d79" = 1.5
  dimension "d80" = 1
  dimension "d81" = 1
  dimension "d91" = 1.5
  dimension "d93" = 1.5
  dimension "d94" = 1
  dimension "d95" = 1.5
  dimension "d96" = 1.5
  dimension "d98" = 1.5
  dimension "d99" = 1.5
  dimension "d100" = 1.5
  dimension "d101" = 1
  constraints: 211 point on circle, 171 symmetric about line, 102 end point, 97 centre point, 37 tangent, 14 equal radius, 13 point on line, 10 coincident, 5 parallel, 3 horizontal, 3 perpendicular, 2 midpoint, 1 concentric, 1 vertical, 72 other
  measures "d71" radial gap between concentric circles of A5 A69
  measures "d72" radius of A67
  measures "d73" distance edge to line of A19 L49
  measures "d74" distance between parallel lines of L25 L50
  measures "d75" distance between parallel lines of L26 L52
  measures "d76" diameter of A71
  measures "d77" radial gap between concentric circles of A41 A70
  measures "d79" radial gap between concentric circles of A72 A30
  measures "d80" distance between parallel lines of L54 L51
  measures "d81" radius of A74
  measures "d91" radial gap between concentric circles of A38 A94
  measures "d93" distance between parallel lines of L64 L63
  measures "d94" radius of A95
  measures "d95" radial gap between concentric circles of A98 A7
  measures "d96" radial gap between concentric circles of A99 A6
  measures "d98" distance between parallel lines of L25 L67
  measures "d99" distance between parallel lines of L23 L68
  measures "d100" distance edge to line of A16 L66
  measures "d101" radius of A100
extrude "押し出し11" cut sketch "肉抜き" against normal blind 2.5 contours A67 A76 A69 A80 L51 A81 A70 A79 A72 L53 A78 L52 A77 L50 A74 L49 A75 L48 | A82 L55 A87 L56 A86 L57 A89 L59 A90 L60 A85 A91 A84 A93 L58 A92 A83 A88 | A98 A105 A99 A104 A103 L67 A102 L68 A100 L65 A101 | A110 A113 L75 A112 L78 A114 L77 A115 A116 A111 A117 | A122 A125 L81 A124 L84 A126 L83 A127 A128 A123 A129 | L90 A141 A140 A138 A139 A137 A136 L88 A135 L87 A134 | A142 L91 A147 L92 A146 L93 A149 L95 A150 L96 A145 A151 A144 A153 L94 A152 A143 A148 | A155 L98 A156 A165 A164 A163 L102 A162 A161 A160 A159 L101 A158 L100 A157 L99 A154 L97
sketch "スケッチ11" plane through (-23, -13, 5.5) normal (0, 1, 0) x (1, 0, 0)
  arc A0 (-40.1624, 81.8203) -> (33.3203, 8.3376) centre (23, 71.5) ccw projected
  circle A1 centre (23, 71.5) radius 64.75
  point P0 (23, 5.5)
  dimension "d109" = 129.5
  constraints: 1 centre point, 1 coincident
  measures "d109" diameter of A1
extrude "押し出し12" cut sketch "スケッチ11" against normal up to surface (2 mm away)
fillet "フィレット6" radius 3 8 edges at (-63.6816, -14, -77.7138) (-62.3716, -14, -83.3879) (-17.3879, -14, -128.3716) (-11.7138, -14, -129.6816) (63.6816, -14, -54.2862) (62.3716, -14, -48.6121) (11.7138, -14, -2.3184) (17.3879, -14, -3.6284)
fillet "フィレット7" radius 1 8 edges at (-62.4813, -14, -49.0104) (-62.9554, -14, -50.8615) (15.1385, -14, -128.9554) (16.9896, -14, -128.4813) (62.4813, -14, -82.9896) (62.9554, -14, -81.1385) (-16.9896, -14, -3.5187) (-15.1385, -14, -3.0446)
